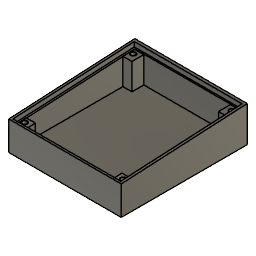
macropad base v0 (Autodesk Fusion 360 design; units mm, degrees)
Autodesk Fusion 360 part; units mm, degrees
note: some values were not read from the file. Chosen so that the rebuilt part matches the saved one: which face or edge a step refers to; which pieces of a blend or face edit are solid.
sketch "Sketch1" plane through (0, 0, 0) normal (0, 0, 1) x (1, 0, 0)
  line L0 (8.8412, 113.5691) -> (103.7772, 113.5691)
  line L1 (103.7772, 113.5691) -> (103.7772, 7.1891)
  line L2 (103.7772, 7.1891) -> (8.8412, 7.1891)
  line L3 (8.8412, 7.1891) -> (8.8412, 113.5691)
  dimension "d1" = 94.936
  dimension "d2" = 106.38
  constraint horizontal L0
  constraint vertical L1
  constraint horizontal L2
  constraint vertical L3
  measures "d1" distance of L0.start L0.end
  measures "d2" distance of L0.start L2.end
extrude "Extrude3" add sketch "Sketch1" along normal blind 30 makes body 1
shell "Shell1" thickness 3.5 removed faces 1 at (40.4866, 42.6491, 30) on bodies 1
sketch "Sketch2" plane through (0, 0, 30) normal (0, 0, 1) x (-1, 0, 0)
  line L0 (-12.3412, -10.6891) -> (-12.3412, -110.0691)
  line L1 (-12.3412, -110.0691) -> (-100.2772, -110.0691)
  line L2 (-100.2772, -110.0691) -> (-100.2772, -10.6891)
  line L3 (-100.2772, -10.6891) -> (-12.3412, -10.6891)
  line L4 (-8.8412, -7.1891) -> (-103.7772, -7.1891)
  line L5 (-103.7772, -7.1891) -> (-103.7772, -113.5691)
  line L6 (-103.7772, -113.5691) -> (-8.8412, -113.5691)
  line L7 (-8.8412, -113.5691) -> (-8.8412, -7.1891)
move_face "MoveFace2" by (70, 0, 0) 1 faces at (40.4866, 42.6491, 0) on bodies 1
move_body "Move1" bodies 1 to x (1, 0, 0) y (0, 1, 0) z (0, 0, 1) at (100, 0, 0)
sketch "Sketch3" plane through (0, 0, 0) normal (0, 0, 1) x (1, 0, 0)
  line L0 (13.9168, 83.2046) -> (104.8528, 83.2046)
  line L1 (104.8528, 83.2046) -> (104.8528, -19.1754)
  line L2 (104.8528, -19.1754) -> (13.9168, -19.1754)
  line L3 (13.9168, -19.1754) -> (13.9168, 83.2046)
  dimension "d21" = 90.936
  dimension "d22" = 102.38
  constraint horizontal L0
  constraint vertical L1
  constraint horizontal L2
  constraint vertical L3
  measures "d21" distance of L0.start L0.end
  measures "d22" distance of L0.start L2.end
extrude "Extrude4" add sketch "Sketch3" along normal blind 4 separate body makes body 2
move_body "Move2" bodies 2 to x (1, 0, 0) y (0, 1, 0) z (0, 0, 1) at (100, 30, 0)
move_body "Move3" bodies 2 to x (1, 0, 0) y (0, 1, 0) z (0, 0, 1) at (-2.6649, -1.4805, 0)
move_face "MoveFace3" by (-10, 0, 0) 1 faces at (141.5639, 77.5975, 4) on bodies 2
move_body "Move4" bodies 2 to x (1, 0, 0) y (0, 1, 0) z (0, 0, 1) at (-0.5, -0.5, 1)
move_body "Move5" bodies 2 to x (1, 0, 0) y (0, 1, 0) z (0, 0, 1) at (-110, 0, 0)
move_body "Move6" bodies 2 to x (1, 0, 0) y (0, 1, 0) z (0, 0, 1) at (0, 0, 25)
move_body "Move7" bodies 2 to x (1, 0, 0) y (0, 1, 0) z (0, 0, 1) at (110, 0, 0)
combine "Combine1" operation cut target body 1 tool bodies 2
sketch "Sketch4" plane through (0, 0, 0) normal (0, 0, 1) x (1, 0, 0)
sketch "Sketch6" plane through (0, 0, 0) normal (0, 0, 1) x (1, 0, 0)
  circle A0 centre (100, 105) radius 2
  dimension "d46" = 4
  measures "d46" diameter of A0
sketch "Sketch9" plane through (0, 0, 0) normal (0, 0, 1) x (1, 0, 0)
  circle A0 centre (13.0966, 36.9251) radius 1.825
  dimension "d61" = 3.65
  measures "d61" diameter of A0
cylinder "CylinderPrimitive2" add diameter 4.5 height 10 placed x (1, 0, 0) y (0, 1, 0) z (0, 0, 1) at (30, 20, 0) separate body makes body 3
extrude "Extrude9" add 1 faces at (30.9164, 19.9724, 10) along direction (0, 0, 1) blind 2.05 on bodies 3 bodies 3
extrude "Extrude10" add 1 faces at (30.9164, 19.9724, 12.05) along direction (0, 0, 1) blind 20 on bodies 3 bodies 3
cylinder "CylinderPrimitive3" add diameter 3.65 height 3.65 placed x (1, 0, 0) y (0, 1, 0) z (0, 0, 1) at (12.9504, 13.5553, 0) separate body makes body 4
extrude "Extrude11" add 1 faces at (13.4295, 13.5259, 3.65) along direction (0, 0, 1) blind 18 on bodies 4 bodies 4
move_body "Move17" bodies 4 to x (1, 0, 0) y (0, 1, 0) z (0, 0, 1) at (15, 5, 20)
move_body "Move18" bodies 4 to x (1, 0, 0) y (0, 1, 0) z (0, 0, 1) at (2.0166, 1.4203, 0)
move_body "Move19" bodies 4 to x (1, 0, 0) y (0, 1, 0) z (0, 0, 1) at (0, 0, -9)
combine "Combine3" operation cut target body 3 tool bodies 4
move_body "Move20" bodies 3 to x (1, 0, 0) y (0, 1, 0) z (0, 0, 1) at (90, 80, 0)
move_body "Move21" bodies 3 to x (1, 0, 0) y (0, 1, 0) z (0, 0, 1) at (0, 0, 2)
move_body "Move22" bodies 3 to x (1, 0, 0) y (0, 1, 0) z (0, 0, 1) at (0, 0, 1.5)
move_body "Move23" bodies 3 to x (1, 0, 0) y (0, 1, 0) z (0, 0, 1) at (-30, 0, -5)
sketch "Sketch14" plane through (0, 0, 0) normal (0, 0, 1) x (1, 0, 0)
  line L0 (15, 25) -> (40, 25)
  line L1 (40, 25) -> (40, 5)
  line L2 (40, 5) -> (15, 5)
  line L3 (15, 5) -> (15, 25)
  constraint horizontal L0
  constraint vertical L1
  constraint horizontal L2
  constraint vertical L3
extrude "Extrude13" add sketch "Sketch14" along normal blind 25 separate body makes body 5
move_body "Move31" bodies 5 to x (1, 0, 0) y (0, 1, 0) z (0, 0, 1) at (15, 90, 0)
move_body "Move32" bodies 5 to x (1, 0, 0) y (0, 1, 0) z (0, 0, 1) at (15, 10, 25)
move_body "Move33" bodies 5 to x (1, 0, 0) y (0, 1, 0) z (0, 0, 1) at (35, 0, 0)
move_body "Move34" bodies 5 to x (1, 0, 0) y (0, 1, 0) z (0, 0, 1) at (0, -15, 0)
move_body "Move35" bodies 5 to x (1, 0, 0) y (0, 1, 0) z (0, 0, 1) at (0, 0, -5)
move_body "Move36" bodies 5 to x (1, 0, 0) y (0, 1, 0) z (0, 0, 1) at (0, 0, -2)
combine "Combine5" operation cut target body 3 tool bodies 5
move_body "Move37" bodies 3 to x (1, 0, 0) y (0, 1, 0) z (0, 0, 1) at (25, 5, 0)
move_body "Move38" bodies 3 to x (1, 0, 0) y (0, 1, 0) z (0, 0, 1) at (0, 0, 5)
extrude "Extrude15" add 1 faces at (117.0286, 105.504, 23) along direction (0, 0, 1) blind 3 on bodies 3 bodies 3
move_body "Move39" bodies 3 to x (1, 0, 0) y (0, 1, 0) z (0, 0, 1) at (0, 0, 0.13)
move_body "Move40" bodies 3 to x (1, 0, 0) y (0, 1, 0) z (0, 0, 1) at (0, 0, 0.585)
move_body "Move41" bodies 3 to x (1, 0, 0) y (0, 1, 0) z (0, 0, 1) at (0, 0, 3)
move_body "Move42" bodies 3 to x (1, 0, 0) y (0, 1, 0) z (0, 0, 1) at (0, 0, -4)
move_body "Move43" bodies 3 to x (1, 0, 0) y (0, 1, 0) z (0, 0, 1) at (0, 2, 0)
move_body "Move44" bodies 3 to x (1, 0, 0) y (0, 1, 0) z (0, 0, 1) at (0, -1, 0)
move_body "Move45" bodies 3 to x (1, 0, 0) y (0, 1, 0) z (0, 0, 1) at (0, -0.41, 0)
move_body "Move46" bodies 3 to x (1, 0, 0) y (0, 1, 0) z (0, 0, 1) at (0.018, 0, 0)
move_body "Move48" bodies 3 to x (1, 0, 0) y (0, 1, 0) z (0, 0, 1) at (-0.3, 0, 0)
move_body "Move49" bodies 3 to x (1, 0, 0) y (0, 1, 0) z (0, 0, 1) at (-0.046, 0, 0)
move_body "Move47" bodies 3 to x (1, 0, 0) y (0, 1, 0) z (0, 0, 1) at (0.25, 0, 0)
move_body "Move52" bodies 3 to x (1, 0, 0) y (0, 1, 0) z (0, 0, 1) at (1.5, 0, 0)
move_body "Move53" bodies 3 to x (1, 0, 0) y (0, 1, 0) z (0, 0, 1) at (0, -0.8, 0)
move_body "Move54" bodies 3 to x (1, 0, 0) y (0, 1, 0) z (0, 0, 1) at (0, 0.1, 0)
move_body "Move55" bodies 3 to x (1, 0, 0) y (0, 1, 0) z (0, 0, 1) at (0, 0.09, 0)
move_body "Move64" bodies 3 to x (1, 0, 0) y (0, 1, 0) z (0, 0, 1) at (-1.45, 0, 0)
move_body "Move65" bodies 3 to x (1, 0, 0) y (0, 1, 0) z (0, 0, 1) at (0, 1.157, 0)
copy_body "CopyPasteBodies3" bodies 3 makes body 6
move_body "Move66" bodies 6 to x (1, 0, 0) y (0, 1, 0) z (0, 0, 1) at (82.5, 0, 0)
move_body "Move67" bodies 6 to x (1, 0, 0) y (0, 1, 0) z (0, 0, 1) at (0.569, 0, 0)
move_body "Move68" bodies 6 to x (1, 0, 0) y (0, 1, 0) z (0, 0, 1) at (0, 0.02, 0)
move_body "Move69" bodies 6 to x (1, 0, 0) y (0, 1, 0) z (0, 0, 1) at (0, -0.04, 0)
copy_body "CopyPasteBodies4" bodies 3 makes body 7
move_body "Move70" bodies 7 to x (1, 0, 0) y (0, 1, 0) z (0, 0, 1) at (0, -91, 0)
move_body "Move71" bodies 7 to x (1, 0, 0) y (0, 1, 0) z (0, 0, 1) at (-0.12, 0, 0)
move_body "Move72" bodies 7 to x (1, 0, 0) y (0, 1, 0) z (0, 0, 1) at (0, -0.498, 0)
copy_body "CopyPasteBodies5" bodies 7 makes body 8
move_body "Move73" bodies 8 to x (1, 0, 0) y (0, 1, 0) z (0, 0, 1) at (82.5, 0, 0)
move_body "Move74" bodies 8 to x (1, 0, 0) y (0, 1, 0) z (0, 0, 1) at (0.58, 0, 0)
move_body "Move75" bodies 8 to x (1, 0, 0) y (0, 1, 0) z (0, 0, 1) at (0, -0.015, 0)
sketch "Sketch15" plane through (0, 0, 0) normal (0, 0, 1) x (1, 0, 0)
  line L0 (20, 30) -> (30, 30)
  line L1 (30, 30) -> (30, 20)
  line L2 (30, 20) -> (20, 20)
  line L3 (20, 20) -> (20, 30)
  constraint horizontal L0
  constraint vertical L1
  constraint horizontal L2
  constraint vertical L3
extrude "Extrude16" add sketch "Sketch15" along normal blind 2 separate body makes body 9
extrude "Extrude17" add 1 faces at (23.3333, 26.6667, 2) along direction (0, 0, 1) blind 3 on bodies 9 bodies 9
move_body "Move76" bodies 9 to x (1, 0, 0) y (0, 1, 0) z (0, 0, 1) at (110, 0, 0)
move_body "Move77" bodies 9 to x (1, 0, 0) y (0, 1, 0) z (0, 0, 1) at (-20, 80, 0)
move_body "Move78" bodies 9 to x (1, 0, 0) y (0, 1, 0) z (0, 0, 1) at (0, 0, 5)
move_body "Move79" bodies 9 to x (1, 0, 0) y (0, 1, 0) z (0, 0, 1) at (0, 0, -2)
copy_body "CopyPasteBodies6" bodies 9 makes body 10
copy_body "CopyPasteBodies7" bodies 10 makes body 11
copy_body "CopyPasteBodies8" bodies 10 makes body 12
move_body "Move80" bodies 11 to x (1, 0, 0) y (0, 1, 0) z (0, 0, 1) at (83.069, 0, 0)
move_body "Move81" bodies 10 to x (1, 0, 0) y (0, 1, 0) z (0, 0, 1) at (0, -91.498, 0)
move_body "Move82" bodies 12 to x (1, 0, 0) y (0, 1, 0) z (0, 0, 1) at (83.08, -91.498, 0)
extrude "Extrude18" add 1 faces at (113.3333, 106.6667, 8) along direction (0, 0, 1) blind 5 on bodies 9 bodies 1 6 7 8 10 11 12 9 3
extrude "Extrude19" add 1 faces at (196.4023, 106.6667, 8) along direction (0, 0, 1) blind 5 on bodies 11 bodies 1 7 8 10 12 11 6
extrude "Extrude20" add 1 faces at (113.3333, 15.1687, 8) along direction (0, 0, 1) blind 5 on bodies 10 bodies 1 8 12 10 7
extrude "Extrude21" add 1 faces at (196.4133, 15.1687, 8) along direction (0, 0, 1) blind 5 on bodies 12 bodies 1 12 8
extrude "Extrude22" add 1 faces at (115.938, 101.3145, 13) along direction (0, 0, 1) blind 10 on bodies 1 bodies 1
extrude "Extrude23" add 1 faces at (115.938, 101.3145, 23) along direction (0, 0, 1) blind 2.7 on bodies 1 bodies 1
extrude "Extrude24" add 1 faces at (197.005, 101.2993, 13) along direction (0, 0, 1) blind 10 on bodies 1 bodies 1
extrude "Extrude25" add 1 faces at (197.005, 101.2993, 23) along direction (0, 0, 1) blind 2.7 on bodies 1 bodies 1
extrude "Extrude26" add 1 faces at (193.9473, 14.605, 13) along direction (0, 0, 1) blind 12.75 on bodies 1 bodies 1
extrude "Extrude27" add 1 faces at (119.034, 14.61, 13) along direction (0, 0, 1) blind 12.7 on bodies 1 bodies 1
draft "Draft1" angle 3 neutral plane through (110.7519, 111.2241, 26) pull (0, -1, 0) 1 faces at (171.4354, 112.7874, 30) on bodies 1
draft "Draft2" angle 3 neutral plane through (108.8412, 110.0691, 0) pull (0, -1, 0) 1 faces at (141.5937, 9.4591, 26) on bodies 1
draft "Draft3" angle 3 neutral plane through (120, 100, 8) pull (0, -1, 0) 1 faces at (119.034, 14.61, 25.7) on bodies 1
draft "Draft4" angle 3 neutral plane through (120, 100, 8) pull (0, -1, 0) 1 faces at (116.8806, 15.143, 25.715) on bodies 1
draft "Draft5" angle 3 neutral plane through (200.2772, 100, 23) pull (0, -1, 0) 1 faces at (199.9606, 15.128, 25.715) on bodies 1
draft "Draft6" angle 3 neutral plane through (200.2772, 100, 23) pull (0, -1, 0) 1 faces at (193.9473, 14.605, 25.75) on bodies 1
extrude "Extrude14" [suppressed]
sketch "Sketch13" plane through (0, 0, 0) normal (0, 0, 1) x (1, 0, 0)
  line L0 (21.934, 44.5534) -> (28.1029, 44.5534)
  line L1 (28.1029, 44.5534) -> (28.1029, 40.4408)
  line L2 (28.1029, 40.4408) -> (21.934, 40.4408)
  line L3 (21.934, 40.4408) -> (21.934, 44.5534)
  constraint horizontal L0
  constraint vertical L1
  constraint horizontal L2
  constraint vertical L3
extrude "Extrude12" [suppressed]
move_body "Move24" [suppressed]
move_body "Move25" [suppressed]
move_body "Move26" [suppressed]
move_body "Move27" [suppressed]
move_body "Move28" [suppressed]
move_body "Move29" [suppressed]
move_body "Move30" [suppressed]
combine "Combine4" [suppressed]
sketch "Sketch7" plane through (0, 0, 0) normal (0, 1, 0) x (1, 0, 0)
  circle A0 centre (20, -20) radius 1.825
  dimension "d49" = 3.65
  measures "d49" diameter of A0
sketch "Sketch8" plane through (0, 0, 0) normal (0, 0, 1) x (1, 0, 0)
  circle A0 centre (20, 50) radius 1.825
  dimension "d58" = 3.65
  measures "d58" diameter of A0
extrude "Extrude7" [suppressed]
extrude "Extrude2" [suppressed]
extrude "Extrude1" [suppressed]
hole "Hole1" [suppressed]
moveface "MoveFace1" [suppressed]
equation "d33 = mm"
